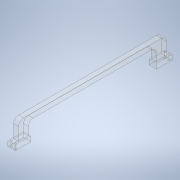
# Autodesk Inventor part: IndexRailOutSides
Saved by Autodesk Inventor 2022 (Build 260153000, 153)
## iProperties
Created: 2022-01-13
Part Number: IndexRailOutSides
Material: Polycarbonate, Clear
Document SubType Name: Modeling
Designer: tagaz
Density: 1.2 g/cm^3
Appearance: Polycarbonate - Clear
Author: tagaz
Autodesk Inventor part; units mm, degrees
ref_plane "YZ Plane" through (0, 0, 0) normal (1, 0, 0) x (0, 1, 0)
ref_plane "XZ Plane" through (0, 0, 0) normal (0, 1, 0) x (-1, 0, 0)
ref_plane "XY Plane" through (0, 0, 0) normal (0, 0, 1) x (1, 0, 0)
sketch "Sketch1" plane through (0, 0, 0) normal (1, 0, 0) x (0, 1, 0)
  line L0 (0, 0) -> (33.909, 0)
  line L1 (59.309, 0) -> (59.309, 12.7)
  line L2 (46.609, 25.4) -> (0, 25.4)
  line L3 (0, 25.4) -> (0, 0)
  line L4 (46.609, -12.7) -> (46.609, -317.5)
  line L5 (59.309, -342.9) -> (59.309, 12.7)
  line L6 (46.609, -355.6) -> (0, -355.6)
  line L7 (0, -355.6) -> (0, -330.2)
  line L8 (0, -330.2) -> (33.909, -330.2)
  arc A0 (59.309, 12.7) -> (46.609, 25.4) centre (46.609, 12.7) ccw
  arc A1 (46.609, -12.7) -> (33.909, 0) centre (33.909, -12.7) ccw
  arc A2 (33.909, -330.2) -> (46.609, -317.5) centre (33.909, -317.5) ccw
  arc A3 (46.609, -355.6) -> (59.309, -342.9) centre (46.609, -342.9) ccw
  dimension "d5" = 25.4
  dimension "d6" = 12.7
  dimension "d7" = 12.7
  dimension "d8" = 12.7
  dimension "d9" = 381
  dimension "d10" = 25.4
  dimension "d11" = 59.309
  dimension "d15" = 59.309
  constraints: 18 end point, 8 point on circle, 8 tangent, 4 centre point, 4 parallel, 2 equal radius, 2 horizontal, 2 perpendicular
  measures "d5" distance of L6.end L7.end
  measures "d6" radius of A0
  measures "d7" radius of A1
  measures "d8" distance between parallel lines of L4 L5
  measures "d9" distance between parallel lines of L2 L6
  measures "d10" distance between parallel lines of L0 L2
  measures "d11" distance between parallel lines of L5 L3
  measures "d15" distance between parallel lines of L5 L7
extrude "Extrusion1" add sketch "Sketch1" along normal mid plane 12.7
sketch "Sketch2" plane through (-6.35, 0, 0) normal (0, -1, 0) x (1, 0, 0)
  line L0 (0, -355.6) -> (12.7, -355.6) projected
  line L1 (0, -330.2) -> (12.7, -330.2) projected
  line L2 (12.7, -355.6) -> (0, -355.6)
  line L3 (0, -355.6) -> (0, -330.2)
  line L4 (0, -330.2) -> (12.7, -330.2)
  line L5 (12.7, -330.2) -> (12.7, -355.6)
  line L6 (-3.175, -327.025) -> (15.875, -327.025)
  line L7 (15.875, -327.025) -> (15.875, -358.775)
  line L8 (-3.175, -358.775) -> (-3.175, -327.025)
  line L9 (12.7, -342.9) -> (0, -342.9) projected
  line L10 (-3.175, -327.025) -> (15.875, -358.775) construction
  line L11 (15.875, -327.025) -> (-3.175, -358.775) construction
  line L12 (15.875, -364.49) -> (15.875, -358.775)
  line L13 (-3.175, -358.775) -> (-3.175, -364.49)
  line L14 (-3.175, -367.03) -> (15.875, -367.03)
  line L15 (15.875, -367.03) -> (15.875, -364.49)
  line L16 (-3.175, -364.49) -> (-3.175, -367.03)
  circle A0 centre (1.27, -362.692) radius 2.54
  line L17 (6.35, -367.03) -> (6.35, -357.004) construction
  circle A1 centre (11.43, -362.692) radius 2.54
  line L18 (42.8308, -165.1) -> (-55.1073, -165.1) construction
  line L19 (0, 25.4) -> (12.7, 25.4)
  line L20 (0, 0) -> (12.7, 0)
  line L21 (12.7, 25.4) -> (0, 25.4)
  line L22 (0, 25.4) -> (0, 0)
  line L23 (0, 0) -> (12.7, 0)
  line L24 (12.7, 0) -> (12.7, 25.4)
  line L25 (-3.175, -3.175) -> (15.875, -3.175)
  line L26 (15.875, -3.175) -> (15.875, 28.575)
  line L27 (-3.175, 28.575) -> (-3.175, -3.175)
  line L28 (12.7, 12.7) -> (0, 12.7)
  line L29 (-3.175, -3.175) -> (15.875, 28.575) construction
  line L30 (15.875, -3.175) -> (-3.175, 28.575) construction
  line L31 (15.875, 34.29) -> (15.875, 28.575)
  line L32 (-3.175, 28.575) -> (-3.175, 34.29)
  line L33 (-3.175, 36.83) -> (15.875, 36.83)
  line L34 (15.875, 36.83) -> (15.875, 34.29)
  line L35 (-3.175, 34.29) -> (-3.175, 36.83)
  circle A2 centre (1.27, 32.492) radius 2.54
  line L36 (6.35, 36.83) -> (6.35, 26.804) construction
  circle A3 centre (11.43, 32.492) radius 2.54
  point P0 (0, 25.4)
  point P1 (12.7, 25.4)
  point P2 (6.35, -342.9)
  point P3 (6.35, 12.7)
  dimension "d16" = 19.05
  dimension "d17" = 31.75
  dimension "d27" = 5.08
  dimension "d28" = 4.445
  constraints: 68 end point, 22 symmetric about line, 6 midpoint, 5 parallel, 4 centre point, 4 horizontal, 3 perpendicular, 2 point on line, 1 vertical, 3 other
  measures "d16" distance of L7.end L8.start
  measures "d17" distance of L6.end L7.end
  measures "d27" diameter of A0
  measures "d28" distance from line of L13 A0.centre
extrude "Extrusion2" add sketch "Sketch2" against normal blind 12.7
body "Solid1"
